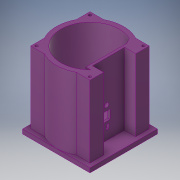
# Autodesk Inventor part: 000.201 - Станина
Saved by Autodesk Inventor 2019 (Build 230136000, 136)
## iProperties
Created: 2020-03-17
Part Number: 000.201 - Станина
Material: Пластик АБС
Document SubType Name: Modeling
Designer: Петров Иван
Density: 1.06 g/cm^3
Appearance: Гладкий — пурпурный
Mass: 1198.69 g
Surface Area: 2238.2 cm^2
Volume: 1130.84 cm^3
Author: Петров Иван
Autodesk Inventor part; units mm, degrees
ref_plane "YZ Plane" through (0, 0, 0) normal (1, 0, 0) x (0, 1, 0)
ref_plane "XZ Plane" through (0, 0, 0) normal (0, 1, 0) x (-1, 0, 0)
ref_plane "XY Plane" through (0, 0, 0) normal (0, 0, 1) x (1, 0, 0)
sketch "Эскиз1" plane through (0, 0, 0) normal (0, 1, 0) x (-1, 0, 0)
  line L0 (-75, 75) -> (75, 75)
  line L1 (75, 75) -> (75, -75)
  line L2 (75, -75) -> (-75, -75)
  line L3 (-75, -75) -> (-75, 75)
  line L4 (-75, 75) -> (75, -75) construction
  line L5 (75, 75) -> (-75, -75) construction
  point P0 (0, 0)
  dimension "d0" = 150
  dimension "d1" = 150
  constraints: 12 end point, 2 midpoint, 2 parallel, 1 horizontal, 1 perpendicular
  measures "d0" distance of L1.end L2.end
  measures "d1" distance of L0.end L1.end
extrude "Выдавливание1" add sketch "Эскиз1" along normal blind 10
sketch "Эскиз2" plane through (0, 10, 0) normal (0, 1, 0) x (1, 0, 0)
  circle A0 centre (0, 0) radius 75
  circle A1 centre (0, 0) radius 65
  dimension "d4" = 150
  dimension "d5" = 130
  constraints: 2 centre point, 2 coincident
  measures "d4" diameter of A0
  measures "d5" diameter of A1
extrude "Выдавливание2" add sketch "Эскиз2" along normal blind 160
sketch "Эскиз3" plane through (0, 10, 0) normal (0, 1, 0) x (1, 0, 0)
  line L0 (0, 0) -> (-53.033, -53.033)
  arc A0 (-75, 0) -> (0, -75) centre (0, 0) ccw projected
  line L1 (0, 0) -> (75, 0) construction
  line L2 (-53.033, -53.033) -> (-66.033, -53.033)
  line L3 (-66.033, -53.033) -> (-66.033, -66.033)
  line L4 (-66.033, -66.033) -> (-53.033, -66.033)
  line L5 (-53.033, -66.033) -> (-53.033, -53.033)
  line L6 (-53.033, -66.033) -> (-35.5618, -66.033)
  line L7 (-66.033, -53.033) -> (-66.033, -35.5618)
  arc A1 (-66.033, -35.5618) -> (-35.5618, -66.033) centre (0, 0) ccw
  circle A2 centre (-59.533, -59.533) radius 3
  dimension "d8" = 135
  dimension "d9" = 13
  dimension "d10" = 13
  dimension "d11" = 6
  dimension "d12" = 6.5
  dimension "d13" = 6.5
  constraints: 16 end point, 6 point on circle, 3 horizontal, 2 centre point, 2 parallel, 2 perpendicular, 1 equal length
  measures "d8" angle of L0 L1
  measures "d9" distance of L4.end L3.end
  measures "d10" distance of L3.end L2.end
  measures "d11" diameter of A2
  measures "d12" distance from line of L3 A2.centre
  measures "d13" distance from line of L4 A2.centre
extrude "Выдавливание3" add sketch "Эскиз3" along normal up to surface (160 mm away)
pattern_circular "Круговой массив1" count 4 over 360 about axis through (0, 10, 0) along (0, 1, 0) of "Выдавливание3"
sketch "Эскиз5" plane through (0, 170, 0) normal (0, 1, 0) x (1, 0, 0)
  line L0 (75, 0) -> (75, 75) projected
  line L1 (75, 35.8218) -> (45, 35.8218)
  line L2 (45, 35.8218) -> (45, -35.5618)
  line L3 (45, -35.5618) -> (75, -35.5618)
  line L4 (75, -35.5618) -> (75, 35.8218)
  point P0 (0, 0)
  dimension "d21" = 30
  constraints: 8 end point, 2 parallel, 1 horizontal, 1 perpendicular, 1 point on line
  measures "d21" distance of L3.end L2.end
extrude "Выдавливание5" cut sketch "Эскиз5" against normal up to surface (160 mm away)
sketch "Эскиз6" plane through (0, 170, 0) normal (0, 1, 0) x (1, 0, 0)
  line L0 (66.033, 66.033) -> (66.033, 35.8218) projected
  line L1 (66.033, 35.8218) -> (36.033, 35.8218)
  line L2 (36.033, 35.8218) -> (36.033, 45.8218)
  line L3 (36.033, 45.8218) -> (66.033, 45.8218)
  line L4 (66.033, 45.8218) -> (66.033, 35.8218)
  arc A0 (54.2384, 35.8218) -> (54.4092, -35.5618) centre (0, 0) ccw projected
  line L5 (36.033, 45.8218) -> (46.6128, 45.8218)
  line L6 (66.033, -35.5618) -> (66.033, -66.033) projected
  line L7 (66.033, -35.5618) -> (36.033, -35.5618)
  line L8 (36.033, -35.5618) -> (36.033, -45.5618)
  line L9 (36.033, -45.5618) -> (66.033, -45.5618)
  line L10 (66.033, -45.5618) -> (66.033, -35.5618)
  line L11 (36.033, 45.8218) -> (41.033, 45.8218)
  line L12 (41.033, 45.8218) -> (41.033, -45.5618)
  line L13 (41.033, -45.5618) -> (36.033, -45.5618)
  line L14 (36.033, -45.5618) -> (36.033, 45.8218)
  dimension "d24" = 30
  dimension "d25" = 10
  dimension "d26" = 30
  dimension "d27" = 10
  dimension "d28" = 5
  constraints: 26 end point, 6 parallel, 4 horizontal, 3 perpendicular, 1 point on line
  measures "d24" distance of L2.end L3.end
  measures "d25" distance of L1.end L2.end
  measures "d26" distance of L9.end L8.end
  measures "d27" distance of L8.end L7.end
  measures "d28" distance of L12.end L13.end
extrude "Выдавливание6" add sketch "Эскиз6" against normal up to surface (160 mm away) contours L0 L1 A0 L3 | L1 L12 L3 A0 | L12 L7 L14 L1 | L1 L2 L3 L12 | L9 L12 L7 A0 | A0 L7 L6 L9 | L12 L9 L8 L7
sketch "Эскиз7" plane through (41.033, 170, 35.5618) normal (1, 0, 0) x (0, 0, -1)
  point P0 (35.5618, -170)
sketch "Эскиз8" plane through (41.033, 170, 35.5618) normal (1, 0, 0) x (0, 0, -1)
  circle A0 centre (31.3816, -91.5) radius 2.1
  line L0 (33.0222, -106.4854) -> (32.894, -106.0661)
  arc A1 (33.0222, -106.4854) -> (33.2588, -106.8521) centre (33.7873, -106.2515) ccw
  line L1 (34.1201, -107.61) -> (33.2588, -106.8521)
  line L2 (34.3916, -117.7894) -> (34.3916, -108.2106)
  arc A2 (34.3916, -108.2106) -> (34.1201, -107.61) centre (33.5916, -108.2106) ccw
  arc A3 (34.1201, -118.39) -> (34.3916, -117.7894) centre (33.5916, -117.7894) ccw
  line L3 (33.2588, -119.1479) -> (34.1201, -118.39)
  line L4 (32.894, -119.9339) -> (33.0222, -119.5146)
  arc A4 (33.2588, -119.1479) -> (33.0222, -119.5146) centre (33.7873, -119.7485) ccw
  arc A5 (32.129, -120.5) -> (32.894, -119.9339) centre (32.129, -119.7) ccw
  line L5 (29.6416, -120.5) -> (32.129, -120.5)
  arc A6 (28.8416, -119.7) -> (29.6416, -120.5) centre (29.6416, -119.7) ccw
  line L6 (28.8416, -106.3) -> (28.8416, -119.7)
  arc A7 (29.6416, -105.5) -> (28.8416, -106.3) centre (29.6416, -106.3) ccw
  line L7 (32.129, -105.5) -> (29.6416, -105.5)
  arc A8 (32.894, -106.0661) -> (32.129, -105.5) centre (32.129, -106.3) ccw
  line L8 (34.2451, -137.4464) -> (33.688, -138.0036)
  line L9 (32.6416, -138.15) -> (33.3345, -138.15)
  arc A9 (33.3345, -138.15) -> (33.688, -138.0036) centre (33.3345, -137.65) ccw
  arc A10 (32.1416, -137.65) -> (32.6416, -138.15) centre (32.6416, -137.65) ccw
  line L10 (32.1416, -131.15) -> (32.1416, -137.65)
  arc A11 (32.6416, -130.65) -> (32.1416, -131.15) centre (32.6416, -131.15) ccw
  line L11 (33.3345, -130.65) -> (32.6416, -130.65)
  line L12 (33.688, -130.7964) -> (34.2451, -131.3536)
  arc A12 (33.688, -130.7964) -> (33.3345, -130.65) centre (33.3345, -131.15) ccw
  arc A13 (34.3916, -131.7071) -> (34.2451, -131.3536) centre (33.8916, -131.7071) ccw
  line L13 (34.3916, -142.5) -> (34.3916, -62.5)
  line L14 (28.8416, -113) -> (34.3916, -113)
  line L15 (24.1166, -123) -> (39.1166, -123)
  line L16 (39.1166, -123) -> (39.1166, -103)
  line L17 (39.1166, -103) -> (24.1166, -103)
  line L18 (24.1166, -103) -> (24.1166, -123)
  line L19 (24.1166, -123) -> (39.1166, -103) construction
  line L20 (39.1166, -123) -> (24.1166, -103) construction
  line L21 (30.3345, -139.4) -> (36.3345, -139.4)
  line L22 (36.3345, -139.4) -> (36.3345, -129.4)
  line L23 (36.3345, -129.4) -> (30.3345, -129.4)
  line L24 (30.3345, -129.4) -> (30.3345, -139.4)
  line L25 (30.3345, -139.4) -> (36.3345, -129.4) construction
  line L26 (36.3345, -139.4) -> (30.3345, -129.4) construction
  circle A14 centre (31.3816, -91.5) radius 5
  circle A15 centre (31.3816, -91.5) radius 2.1
  line L27 (33.0222, -106.4854) -> (32.894, -106.0661)
  arc A16 (33.0222, -106.4854) -> (33.2588, -106.8521) centre (33.7873, -106.2515) ccw
  line L28 (34.1201, -107.61) -> (33.2588, -106.8521)
  line L29 (34.3916, -117.7894) -> (34.3916, -108.2106)
  arc A17 (34.3916, -108.2106) -> (34.1201, -107.61) centre (33.5916, -108.2106) ccw
  arc A18 (34.1201, -118.39) -> (34.3916, -117.7894) centre (33.5916, -117.7894) ccw
  line L30 (33.2588, -119.1479) -> (34.1201, -118.39)
  line L31 (32.894, -119.9339) -> (33.0222, -119.5146)
  arc A19 (33.2588, -119.1479) -> (33.0222, -119.5146) centre (33.7873, -119.7485) ccw
  arc A20 (32.129, -120.5) -> (32.894, -119.9339) centre (32.129, -119.7) ccw
  line L32 (29.6416, -120.5) -> (32.129, -120.5)
  arc A21 (28.8416, -119.7) -> (29.6416, -120.5) centre (29.6416, -119.7) ccw
  line L33 (28.8416, -106.3) -> (28.8416, -119.7)
  arc A22 (29.6416, -105.5) -> (28.8416, -106.3) centre (29.6416, -106.3) ccw
  line L34 (32.129, -105.5) -> (29.6416, -105.5)
  arc A23 (32.894, -106.0661) -> (32.129, -105.5) centre (32.129, -106.3) ccw
  line L35 (34.2451, -137.4464) -> (33.688, -138.0036)
  line L36 (32.6416, -138.15) -> (33.3345, -138.15)
  arc A24 (33.3345, -138.15) -> (33.688, -138.0036) centre (33.3345, -137.65) ccw
  arc A25 (32.1416, -137.65) -> (32.6416, -138.15) centre (32.6416, -137.65) ccw
  line L37 (32.1416, -131.15) -> (32.1416, -137.65)
  arc A26 (32.6416, -130.65) -> (32.1416, -131.15) centre (32.6416, -131.15) ccw
  line L38 (33.3345, -130.65) -> (32.6416, -130.65)
  line L39 (33.688, -130.7964) -> (34.2451, -131.3536)
  arc A27 (33.688, -130.7964) -> (33.3345, -130.65) centre (33.3345, -131.15) ccw
  arc A28 (34.3916, -131.7071) -> (34.2451, -131.3536) centre (33.8916, -131.7071) ccw
  line L40 (34.3916, -142.5) -> (34.3916, -62.5)
  line L41 (28.8416, -113) -> (34.3916, -113)
  line L42 (24.1166, -123) -> (39.1166, -123)
  line L43 (39.1166, -123) -> (39.1166, -103)
  line L44 (39.1166, -103) -> (24.1166, -103)
  line L45 (24.1166, -103) -> (24.1166, -123)
  line L46 (24.1166, -123) -> (39.1166, -103) construction
  line L47 (39.1166, -123) -> (24.1166, -103) construction
  line L48 (30.3345, -139.4) -> (36.3345, -139.4)
  line L49 (36.3345, -139.4) -> (36.3345, -129.4)
  line L50 (36.3345, -129.4) -> (30.3345, -129.4)
  line L51 (30.3345, -129.4) -> (30.3345, -139.4)
  line L52 (30.3345, -139.4) -> (36.3345, -129.4) construction
  line L53 (36.3345, -139.4) -> (30.3345, -129.4) construction
  circle A29 centre (31.3816, -91.5) radius 5
  point P0 (35.5618, -170)
  point P1 (31.6166, -113)
  point P2 (33.3345, -134.4)
  point P3 (31.6166, -113)
  point P4 (33.3345, -134.4)
  dimension "d31" = 15
  dimension "d32" = 20
  dimension "d33" = 6
  dimension "d34" = 10
  dimension "d35" = 10
  dimension "d36" = 15
  dimension "d37" = 20
  dimension "d38" = 6
  dimension "d39" = 10
  dimension "d40" = 10
  constraints: 108 end point, 52 point on circle, 30 centre point, 12 midpoint, 8 parallel, 6 perpendicular, 4 horizontal, 2 coincident, 2 point on line
  measures "d31" distance of L17.end L16.end
  measures "d32" distance of L16.end L15.end
  measures "d33" distance of L23.end L22.end
  measures "d34" distance of L22.end L21.end
  measures "d35" diameter of A14
  measures "d36" distance of L44.end L43.end
  measures "d37" distance of L43.end L42.end
  measures "d38" distance of L50.end L49.end
  measures "d39" distance of L49.end L48.end
  measures "d40" diameter of A29
extrude "Выдавливание7" cut sketch "Эскиз8" against normal blind 10 contours A0 | A1 L1 A2 L2 L14 L6 A7 L7 A8 L0 | L0 A8 L7 A7 L6 A6 L5 A5 L4 A4 L3 A3 L13 L15 L18 L17 A2 L1 A1 | L13 L17 L16 L15 L2 | L2 A3 L3 A4 L4 A5 L5 A6 L6 L14 | L21 L24 L23 L13 | L13 L23 L22 L21 | A14 L13 | L13 A14
chamfer "Фаска1" distance 20.818 distance2 10.068 1 edges at (46.1017, 90, -45.8218) measured on face at (45.7479, 90, -46.175)
